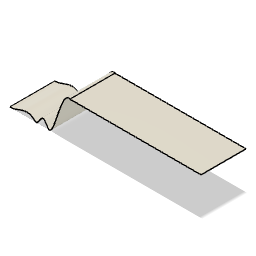
paper v2 (Autodesk Fusion 360 design; units mm, degrees)
Autodesk Fusion 360 part; units mm, degrees
sketch "Sketch1" plane through (0, 0, 0) normal (1, 0, 0) x (0, 0, -1)
  line L0 (0, 0) -> (120, 0)
  line L1 (120, 0) -> (120, 1)
  line L2 (120, 1) -> (0, 1)
  line L3 (0, 1) -> (0, 0)
  dimension "d1" = 120
  dimension "d2" = 1
  constraint horizontal L0
  constraint vertical L1
  constraint horizontal L2
  constraint vertical L3
  constraint coincident L0.start L3.end
  measures "d1" distance of L0.start L0.end
  measures "d2" distance of L0.start L2.end
sketch "Sketch2" plane through (0, 0, 0) normal (0, 0, 1) x (1, 0, 0)
  line L0 (0, 0) -> (-350, 0)
  spline S0 degree 5 poles (-350, 0) (-350.8271, 0.4587) (-352.4933, 1.0797) (-355.0292, 1.1216) (-358.4834, -0.6039) (-362.9205, -5.695) (-367.4691, -13.5915) (-372.1125, -24.0179) (-376.8222, -36.4948) (-381.5546, -50.2909) (-386.2473, -64.3452) (-390.8275, -77.4151) (-395.2241, -88.2647) (-399.3789, -95.8428) (-403.2569, -99.458) (-406.8592, -98.9768) (-410.2319, -94.9687) (-413.4842, -88.9957) (-416.7636, -83.2728) (-420.1972, -79.8916) (-423.8523, -80.2595) (-427.6694, -84.2554) (-431.4759, -90.2056) (-435.0991, -95.877) (-438.4529, -99.195) (-441.6396, -99.1071) (-445.0314, -96.2902) (-449.0787, -92.2979) (-454.1548, -88.876) (-460.3477, -87.0727) (-467.4593, -87.1207) (-475.1186, -88.7395) (-482.8603, -91.3086) (-490.2148, -94.0877) (-496.7975, -96.4244) (-502.3863, -97.9415) (-505.9753, -98.3489) (-508.1562, -98.1745) (-509.3833, -97.8452) (-509.9402, -97.6273) knots 0 0 0 0 0 0 0.028571 0.057143 0.085714 0.114286 0.142857 0.171429 0.2 0.228571 0.257143 0.285714 0.314286 0.342857 0.371429 0.4 0.428571 0.457143 0.485714 0.514286 0.542857 0.571429 0.6 0.628571 0.657143 0.685714 0.714286 0.742857 0.771429 0.8 0.828571 0.857143 0.885714 0.914286 0.942857 0.971429 1 1 1 1 1 1
  point P0 (-377.6352, -39.0751)
  point P1 (-408.1284, -97.0388)
  point P2 (-422.2526, -80.5606)
  point P3 (-438.1423, -98.2158)
  point P4 (-451.0895, -91.1537)
  point P5 (-489.2531, -93.6998)
  dimension "d3" = 350
  constraint coincident L0.start origin
  measures "d3" distance of L0.start L0.end
sweep "Sweep1" add profiles "Sketch1" path "Sketch2" along L0 S0 section 1
